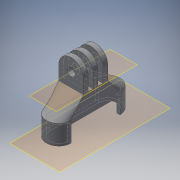
# Autodesk Inventor part: camera_mount_down
Saved by Autodesk Inventor 2018 (Build 220112000, 112)
## iProperties
Created: 2018-01-12
Part Number: camera_mount_down
Material: Generic
Document SubType Name: Modeling
Designer: erwin
Density: 1 g/cm^3
Appearance: Default
Author: erwin
Autodesk Inventor part; units mm, degrees
ref_plane "YZ Plane" through (0, 0, 0) normal (1, 0, 0) x (0, 1, 0)
ref_plane "XZ Plane" through (0, 0, 0) normal (0, 1, 0) x (-1, 0, 0)
ref_plane "XY Plane" through (0, 0, 0) normal (0, 0, 1) x (1, 0, 0)
ref_plane "Work Plane1" through (0, 0, 0) normal (0, 0, 1) x (1, 0, 0)
sketch "Sketch1" plane through (0, 0, 0) normal (0, 0, 1) x (1, 0, 0)
  circle A0 centre (-8.2045, 36.5379) radius 1.5 projected
  circle A1 centre (-8.2045, 6.5379) radius 1.5 projected
  line L0 (-12.2045, 11.5379) -> (-12.2045, 31.5379) projected
  line L1 (-12.2045, 31.5379) -> (-2.2045, 31.5379) projected
  line L2 (-2.2045, 31.5379) -> (-2.2045, 11.5379) projected
  line L3 (-2.2045, 11.5379) -> (-12.2045, 11.5379) projected
  line L4 (9.7955, -5.4621) -> (9.7955, 48.5379) projected
  line L5 (9.7955, 48.5379) -> (-11.2045, 48.5379) projected
  line L6 (-11.2045, 48.5379) -> (-11.2045, 52.2879) projected
  line L7 (-11.2045, 52.2879) -> (-15.7045, 52.2879) projected
  line L8 (-15.7045, 52.2879) -> (-15.7045, 45.5379) projected
  line L9 (-15.7045, 45.5379) -> (-17.9545, 45.5379) projected
  line L10 (-17.9545, 45.5379) -> (-17.9545, -2.4621) projected
  line L11 (-17.9545, -2.4621) -> (-15.7045, -2.4621) projected
  line L12 (-15.7045, -2.4621) -> (-15.7045, -9.2121) projected
  line L13 (-15.7045, -9.2121) -> (-11.2045, -9.2121) projected
  line L14 (-11.2045, -9.2121) -> (-11.2045, -5.4621) projected
  line L15 (-11.2045, -5.4621) -> (9.7955, -5.4621) projected
  line L16 (-15.7045, 6.5379) -> (-15.7045, 36.5379)
  line L17 (-13.7045, 36.5379) -> (-13.7045, 6.5379)
  line L18 (-2.7045, 36.5379) -> (-0.7045, 36.5379)
  line L19 (-2.7045, 6.5379) -> (-0.7045, 6.5379)
  arc A2 (-12.2045, 30.1936) -> (-2.6143, 31.5379) centre (-8.2045, 36.5379) ccw
  arc A3 (-0.7045, 36.5379) -> (-15.7045, 36.5379) centre (-8.2045, 36.5379) ccw
  arc A4 (-10.4958, 31.5379) -> (-5.9132, 31.5379) centre (-8.2045, 36.5379) ccw
  arc A5 (-2.7045, 36.5379) -> (-13.7045, 36.5379) centre (-8.2045, 36.5379) ccw
  arc A6 (-5.9132, 11.5379) -> (-10.4958, 11.5379) centre (-8.2045, 6.5379) ccw
  arc A7 (-13.7045, 6.5379) -> (-2.7045, 6.5379) centre (-8.2045, 6.5379) ccw
  arc A8 (-2.6143, 11.5379) -> (-13.7045, 11.6369) centre (-8.2045, 6.5379) ccw
  arc A9 (-15.7045, 6.5379) -> (-0.7045, 6.5379) centre (-8.2045, 6.5379) ccw
  point P0 (0, 0)
  constraints: 16 point on circle, 8 centre point, 8 end point, 8 point on line, 2 parallel, 1 vertical
extrude "Extrusion1" add sketch "Sketch1" along normal blind 10 contours L16 A3 L18 A5 L17 A7 L19 A9
sketch "Sketch2" plane through (0, 0, 10) normal (0, 0, 1) x (1, 0, 0)
  line L0 (-13.7045, 6.5379) -> (-13.7045, 36.5379) projected
  arc A0 (-2.7045, 36.5379) -> (-13.7045, 36.5379) centre (-8.2045, 36.5379) ccw projected
  line L1 (-2.7045, 36.5379) -> (-0.7045, 36.5379) projected
  arc A1 (-0.7045, 36.5379) -> (-15.7045, 36.5379) centre (-8.2045, 36.5379) ccw projected
  line L2 (-15.7045, 36.5379) -> (-15.7045, 6.5379) projected
  arc A2 (-15.7045, 6.5379) -> (-0.7045, 6.5379) centre (-8.2045, 6.5379) ccw projected
  line L3 (-0.7045, 6.5379) -> (-2.7045, 6.5379) projected
  arc A3 (-13.7045, 6.5379) -> (-2.7045, 6.5379) centre (-8.2045, 6.5379) ccw projected
  line L4 (-0.7045, 36.5379) -> (-0.7045, 6.5379)
  point P0 (0, 0)
  constraints: 2 end point, 1 tangent, 1 vertical
extrude "Extrusion2" add sketch "Sketch2" along normal blind 2
ref_plane "Work Plane2" through (0, 0, 22) normal (0, 0, 1) x (1, 0, 0)
sketch "Sketch3" plane through (0, 0, 22) normal (0, 0, 1) x (1, 0, 0)
  line L0 (-0.7045, 6.5379) -> (-0.7045, 36.5379) projected
  line L1 (-15.7045, 29.0379) -> (-0.7045, 29.0379)
  line L2 (-0.7045, 29.0379) -> (-0.7045, 14.0379)
  line L3 (-0.7045, 14.0379) -> (-15.7045, 14.0379)
  line L4 (-15.7045, 14.0379) -> (-15.7045, 29.0379)
  line L5 (-15.7045, 29.0379) -> (-0.7045, 14.0379) construction
  line L6 (-0.7045, 29.0379) -> (-15.7045, 14.0379) construction
  line L7 (-15.7045, 36.5379) -> (-15.7045, 6.5379) construction
  line L8 (-15.7045, 21.5379) -> (19.8362, 21.5379) construction
  point P0 (0, 0)
  point P1 (-8.2045, 21.5379)
  dimension "d9" = 15
  constraints: 14 end point, 3 midpoint, 2 horizontal, 2 parallel, 1 perpendicular, 1 point on line, 1 other
  measures "d9" distance of L1.end L2.end
loft "Loft1" add profiles "Sketch3" section 1 edges at (-8.2045, 44.0379, 12) (-15.7045, 21.5379, 12) (-8.2045, -0.9621, 12) (-0.7045, 21.5379, 12)
sketch "Sketch4" plane through (-15.7045, 29.0379, 22) normal (0, 0, 1) x (1, 0, 0)
  line L0 (0, -15) -> (0, 0) projected
  line L1 (15, 0) -> (15, -15) projected
  line L2 (0, 0) -> (15, 0)
  line L3 (15, 0) -> (15, -3)
  line L4 (15, -3) -> (0, -3)
  line L5 (0, -3) -> (0, 0)
  line L6 (0, -6) -> (15, -6)
  line L7 (15, -6) -> (15, -9)
  line L8 (15, -9) -> (0, -9)
  line L9 (0, -9) -> (0, -6)
  line L10 (0, -12) -> (15, -12)
  line L11 (15, -12) -> (15, -15)
  line L12 (15, -15) -> (0, -15)
  line L13 (0, -15) -> (0, -12)
  point P0 (15.7045, -29.0379)
  dimension "d14" = 3
  dimension "d17" = 6
  constraints: 24 end point, 2 parallel, 1 horizontal, 1 perpendicular, 1 point on line, 1 vertical, 16 other
  measures "d14" distance of L2.end L3.end
  measures "d17" distance of L3.end L7.end
extrude "Extrusion3" add sketch "Sketch4" along normal blind 16 contours L0 L10 L1 L12 | L0 L6 L1 L8 | L0 L2 L1 L4
sketch "Sketch5" plane through (-15.7045, 14.0379, 22) normal (0, -1, 0) x (1, 0, 0)
  line L0 (15, 8.5) -> (15, 16)
  line L1 (0, 16) -> (15, 16) projected
  line L2 (0, 8.5) -> (0, 16)
  arc A0 (15, 8.5) -> (0, 8.5) centre (7.5, 8.5) ccw
  point P0 (15.7045, -22)
  point P1 (7.5, 16)
  constraints: 4 end point, 3 point on circle, 3 tangent, 1 centre point, 1 midpoint
extrude "Extrusion4" cut sketch "Sketch5" against normal through all
hole "Hole1" at (-8.2045, 14.0379, 30.5) direction (0, 1, 0) diameter 5 end through all
body "Solid1"
